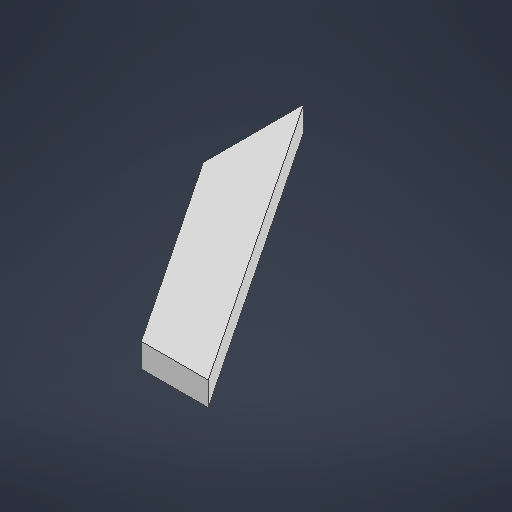
# Autodesk Inventor part: S_2x4x21.633
Saved by Autodesk Inventor 2026 (Build 300175000, 175)
## iProperties
Created: 2025-09-08
Part Number: S_2x4x21.633
Material: Generic
Document SubType Name: Modeling
Designer: trott
Density: 1 g/cm^3
Appearance: Default
Author: trott
Autodesk Inventor part; units mm, degrees
ref_plane "YZ Plane" through (0, 0, 0) normal (1, 0, 0) x (0, 1, 0)
ref_plane "XZ Plane" through (0, 0, 0) normal (0, 1, 0) x (-1, 0, 0)
ref_plane "XY Plane" through (0, 0, 0) normal (0, 0, 1) x (1, 0, 0)
sketch "Sketch1" plane through (0, 0, 0) normal (0, 1, 0) x (-1, 0, 0)
  line L0 (0, 0) -> (-609.6, 0)
  line L1 (-609.6, 0) -> (-914.4, 0)
  line L2 (-914.4, 0) -> (-914.4, 152.4)
  line L3 (-609.6, 0) -> (-914.4, 152.4)
  line L4 (0, 0) -> (0, 304.8)
  line L5 (0, 304.8) -> (-609.6, 0)
  line L6 (-914.4, 0) -> (-914.4, -762)
  line L7 (0, 0) -> (0, -1219.2)
  line L8 (0, -1219.2) -> (-609.6, -1219.2)
  line L9 (-609.6, -1219.2) -> (-914.4, -762)
  line L10 (-914.4, -762) -> (-840.4307, -712.6872)
  line L11 (-609.6, -1219.2) -> (-535.6307, -1169.8872)
  line L12 (0, -1219.2) -> (0, -1130.3)
  line L13 (0, -1130.3) -> (-609.6, -1130.3)
  line L14 (-609.6, -1130.3) -> (-609.6, -1219.2)
  line L15 (-914.4, -762) -> (-825.5, -762)
  line L16 (-825.5, -762) -> (-825.5, 0)
  line L17 (-840.4307, -712.6872) -> (-535.6307, -1169.8872)
  line L18 (-609.6, -1130.3) -> (-609.6, 0)
  line L19 (-825.5, -762) -> (-609.6, -762)
  point P0 (-609.6, -1058.9332)
  point P1 (-807.5555, -762)
  dimension "d0" = 609.6
  dimension "d1" = 304.8
  dimension "d2" = 152.4
  dimension "d3" = 304.8
  dimension "d4" = 762
  dimension "d5" = 1219.2
  dimension "d6" = 609.6
  dimension "d7" = 88.9
  dimension "d8" = 88.9
  dimension "d9" = 88.9
  dimension "d10" = 609.6
  dimension "d11" = 88.9
  constraints: 40 end point, 9 perpendicular, 4 point on line, 1 horizontal, 1 parallel, 1 vertical
  measures "d0" distance of L0.start L0.end
  measures "d1" distance of L0.end L1.end
  measures "d2" distance of L1.end L2.end
  measures "d3" distance of L0.start L4.end
  measures "d4" distance of L1.end L6.end
  measures "d5" distance of L0.start L7.end
  measures "d6" distance of L7.end L8.end
  measures "d7" distance of L6.end L10.end
  measures "d8" distance of L8.end L11.end
  measures "d9" distance of L7.end L12.end
  measures "d10" distance of L12.end L13.end
  measures "d11" distance of L6.end L15.end
extrude "Extrusion1" add sketch "Sketch1" along normal blind 38.1 contours L18 L14 L9 L15 L19 L17
body "Solid1"
